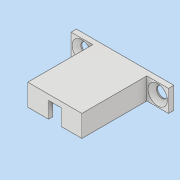
# Autodesk Inventor part: potentiometerMountForePlanes
Saved by Autodesk Inventor 2017 (Build 210142000, 142)
## iProperties
Created: 2016-12-10
Part Number: potentiometerMountForePlanes
Material: ABS Plastic
Document SubType Name: Modeling
Designer: techn
Density: 1.06 g/cm^3
Appearance: Smooth - White
Author: techn
Autodesk Inventor part; units mm, degrees
ref_plane "YZ Plane" through (0, 0, 0) normal (1, 0, 0) x (0, 1, 0)
ref_plane "XZ Plane" through (0, 0, 0) normal (0, 1, 0) x (-1, 0, 0)
ref_plane "XY Plane" through (0, 0, 0) normal (0, 0, 1) x (1, 0, 0)
sketch "Sketch1" plane through (0, 0, 0) normal (0, 0, 1) x (1, 0, 0)
  circle A0 centre (0, 0) radius 1.5875
  circle A1 centre (22.225, 0) radius 1.5875
  line L0 (-3.175, 3.175) -> (25.4, 3.175)
  line L1 (25.4, 3.175) -> (25.4, -3.175)
  line L2 (25.4, -3.175) -> (-3.175, -3.175)
  line L3 (-3.175, -3.175) -> (-3.175, 3.175)
  dimension "d0" = 3.175
  dimension "d1" = 3.175
  dimension "d2" = 22.225
  dimension "d3" = 3.175
  dimension "d4" = 3.175
  dimension "d5" = 3.175
  dimension "d6" = 3.175
  constraints: 8 end point, 2 centre point, 2 parallel, 1 coincident, 1 horizontal, 1 horizontal alignment, 1 perpendicular
  measures "d0" diameter of A0
  measures "d1" diameter of A1
  measures "d2" distance of A1.centre point (0, 0)
  measures "d3" distance from line of point (0, 0) L3
  measures "d4" distance from line of L1 A1.centre
  measures "d5" distance from line of L0 A1.centre
  measures "d6" distance from line of L2 point (0, 0)
extrude "Extrusion1" add sketch "Sketch1" along normal blind 1.5875
sketch "Sketch2" plane through (0, 0, 1.5875) normal (0, 0, 1) x (1, 0, 0)
  circle A0 centre (22.225, 0) radius 1.5875 projected
  circle A1 centre (0, 0) radius 1.5875 projected
  line L0 (25.4, 3.175) -> (-3.175, 3.175) projected
  line L1 (-3.175, 3.175) -> (-3.175, -3.175) projected
  line L2 (-3.175, -3.175) -> (25.4, -3.175) projected
  line L3 (25.4, -3.175) -> (25.4, 3.175) projected
  line L4 (3.175, 3.175) -> (19.05, 3.175)
  line L5 (19.05, 3.175) -> (19.05, -3.175)
  line L6 (19.05, -3.175) -> (3.175, -3.175)
  line L7 (3.175, -3.175) -> (3.175, 3.175)
  dimension "d9" = 15.875
  dimension "d10" = 3.175
  constraints: 8 end point, 2 parallel, 2 point on line, 1 horizontal, 1 perpendicular
  measures "d9" distance between parallel lines of L5 L7
  measures "d10" distance from line of L7 point (0, 0)
extrude "Extrusion2" add sketch "Sketch2" along normal blind 19.05 contours L5 L2 L7 L0
sketch "Sketch3" plane through (-3.175, -3.175, 0) normal (0, -1, 0) x (1, 0, 0)
  line L0 (28.575, 0) -> (0, 0) projected
  line L1 (28.575, 0) -> (28.575, 1.5875) projected
  line L2 (22.225, 1.5875) -> (28.575, 1.5875) projected
  line L3 (22.225, 1.5875) -> (22.225, 20.6375) projected
  line L4 (6.35, 20.6375) -> (22.225, 20.6375) projected
  line L5 (6.35, 1.5875) -> (6.35, 20.6375) projected
  line L6 (0, 1.5875) -> (6.35, 1.5875) projected
  line L7 (0, 0) -> (0, 1.5875) projected
  line L8 (6.35, 1.5875) -> (22.225, 1.5875)
  circle A0 centre (14.2875, 13.0175) radius 6.604
  line L9 (12.4481, 19.3602) -> (12.4481, 20.6375)
  line L10 (16.1269, 19.3602) -> (16.1269, 20.6375)
  point P0 (3.175, 0)
  dimension "d13" = 13.208
  dimension "d14" = 7.62
  constraints: 6 end point, 2 perpendicular, 2 point on circle, 2 point on line, 1 centre point, 1 parallel
  measures "d13" diameter of A0
  measures "d14" distance from line of A0.centre L4
extrude "Extrusion4" cut sketch "Sketch3" against normal blind 4.7625 contours L10 A0 L9 L4 | A0
chamfer "Chamfer1" distance 1.27 angle 45 2 edges at (-1.5875, 0, 1.5875) (20.6375, 0, 1.5875)
body "Solid1"
